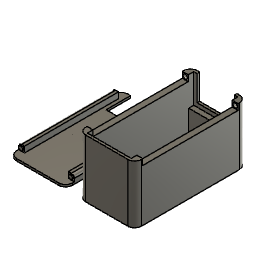
WirelessTouchLight v5 (Autodesk Fusion 360 design; units mm, degrees)
Autodesk Fusion 360 part; units mm, degrees
form "Form1" [no effect]
sketch "Bases" plane through (0, 0, 0) normal (0, 1, 0) x (1, 0, 0)
  line L0 (7.8348, -10.0405) -> (32.8348, -10.0405)
  line L1 (36.8348, -6.0405) -> (36.8348, 51.9595)
  line L2 (32.8348, 55.9595) -> (7.8348, 55.9595)
  line L3 (3.8348, 51.9595) -> (3.8348, -6.0405)
  arc A0 (7.8348, 55.9595) -> (3.8348, 51.9595) centre (7.8348, 51.9595) ccw
  arc A1 (36.8348, 51.9595) -> (32.8348, 55.9595) centre (32.8348, 51.9595) ccw
  arc A2 (32.8348, -10.0405) -> (36.8348, -6.0405) centre (32.8348, -6.0405) ccw
  arc A3 (3.8348, -6.0405) -> (7.8348, -10.0405) centre (7.8348, -6.0405) ccw
  arc A4 (3.8348, -6.0405) -> (7.8348, -10.0405) centre (7.8348, -6.0405) ccw
  arc A5 (32.8348, -10.0405) -> (36.8348, -6.0405) centre (32.8348, -6.0405) ccw
  line L4 (3.8348, 51.9595) -> (3.8348, -6.0405)
  line L5 (36.8348, -6.0405) -> (36.8348, 51.9595)
  line L6 (7.8348, -10.0405) -> (32.8348, -10.0405)
  arc A6 (7.8348, 55.9595) -> (3.8348, 51.9595) centre (7.8348, 51.9595) ccw
  line L7 (32.8348, 55.9595) -> (7.8348, 55.9595)
  arc A7 (36.8348, 51.9595) -> (32.8348, 55.9595) centre (32.8348, 51.9595) ccw
  line L8 (-37.5541, 52.4657) -> (-37.5541, -5.5343)
  arc A8 (-8.5541, -9.5343) -> (-4.5541, -5.5343) centre (-8.5541, -5.5343) ccw
  line L9 (-33.5541, -9.5343) -> (-8.5541, -9.5343)
  line L10 (-8.5541, 56.4657) -> (-33.5541, 56.4657)
  arc A9 (-33.5541, 56.4657) -> (-37.5541, 52.4657) centre (-33.5541, 52.4657) ccw
  arc A10 (-4.5541, 52.4657) -> (-8.5541, 56.4657) centre (-8.5541, 52.4657) ccw
  arc A11 (-37.5541, -5.5343) -> (-33.5541, -9.5343) centre (-33.5541, -5.5343) ccw
  line L11 (-4.5541, -5.5343) -> (-4.5541, 52.4657)
  line L12 (-37.5541, 51.2657) -> (-34.0541, 51.2657)
  line L13 (-34.0541, 51.2657) -> (-34.0541, -4.3343)
  line L14 (-34.0541, -4.3343) -> (-37.5541, -4.3343)
  line L15 (-37.5541, -4.3343) -> (-37.5541, 51.2657)
  line L16 (-4.5541, 51.2657) -> (-8.0541, 51.2657)
  line L17 (-8.0541, 51.2657) -> (-8.0541, -4.3343)
  line L18 (-8.0541, -4.3343) -> (-4.5541, -4.3343)
  line L19 (-4.5541, -4.3343) -> (-4.5541, 51.2657)
  dimension "d14" = 4
  dimension "d15" = 4
  dimension "d16" = 66
  dimension "d18" = 33
  dimension "d31" = 4
  dimension "d32" = 4
  dimension "d33" = 66
  dimension "d34" = 33
  dimension "d35" = 4
  dimension "d36" = 4
  dimension "d37" = 66
  dimension "d38" = 33
  dimension "d45" = 55.6
  dimension "d46" = 3.5
  dimension "d47" = 3.5
  constraint horizontal L0
  constraint vertical L1
  constraint horizontal L2
  constraint vertical L3
  constraint tangent L2 A0
  constraint tangent L3 A0
  constraint tangent L1 A1
  constraint tangent L2 A1
  constraint tangent L0 A2
  constraint tangent L1 A2
  constraint equal A1 A2
  constraint tangent L0 A3
  constraint tangent L3 A3
  constraint equal A1 A3
  constraint horizontal L6
  constraint vertical L5
  constraint horizontal L7
  constraint vertical L4
  constraint tangent A6 L7
  constraint tangent L4 A6
  constraint tangent L5 A7
  constraint tangent L7 A7
  constraint tangent A5 L6
  constraint tangent A5 L5
  constraint equal A5 A7
  constraint tangent A4 L6
  constraint tangent A4 L4
  constraint equal A4 A7
  constraint horizontal L9
  constraint vertical L11
  constraint horizontal L10
  constraint vertical L8
  constraint tangent L10 A9
  constraint tangent L8 A9
  constraint tangent A10 L11
  constraint tangent L10 A10
  constraint tangent A8 L9
  constraint tangent A8 L11
  constraint equal A8 A10
  constraint tangent L9 A11
  constraint tangent L8 A11
  constraint equal A10 A11
  constraint horizontal L12
  constraint vertical L13
  constraint horizontal L14
  constraint vertical L15
  constraint coincident L8 L12.start
  constraint midpoint L8 L15
  constraint horizontal L16
  constraint vertical L17
  constraint horizontal L18
  constraint vertical L19
  constraint collinear L12 L16
  constraint collinear L14 L18
  constraint collinear L11 L19
  measures "d14" radius of A0
  measures "d15" radius of A1
  measures "d16" distance of L0 L2
  measures "d18" distance of L1 L3
  measures "d31" radius of A6
  measures "d32" radius of A7
  measures "d33" distance of L6 L7
  measures "d34" distance of L4 L5
  measures "d35" radius of A9
  measures "d36" radius of A10
  measures "d37" distance of L9 L10
  measures "d38" distance of L8 L11
  measures "d45" distance of L12.end L13.end
  measures "d46" distance of L12.start L12.end
  measures "d47" distance of L16.start L16.end
extrude "WirelessTouchLight Box" add sketch "Bases" along normal blind 34.25 contours L0 L1 L2 L3 A0 A1 A2 A3 A4 A5 L4 L5 L6 A6 L7 A7 makes body 1
sketch "TopBox" plane through (0, 34.25, 0) normal (0, 1, 0) x (-1, 0, 0)
  arc A0 (-3.8348, 6.0405) -> (-7.8348, 10.0405) centre (-7.8348, 6.0405) ccw
  line L0 (-7.8348, 10.0405) -> (-32.8348, 10.0405)
  arc A1 (-32.8348, 10.0405) -> (-36.8348, 6.0405) centre (-32.8348, 6.0405) ccw
  line L1 (-36.8348, 6.0405) -> (-36.8348, -51.9595)
  arc A2 (-36.8348, -51.9595) -> (-32.8348, -55.9595) centre (-32.8348, -51.9595) ccw
  line L2 (-32.8348, -55.9595) -> (-7.8348, -55.9595)
  arc A3 (-7.8348, -55.9595) -> (-3.8348, -51.9595) centre (-7.8348, -51.9595) ccw
  line L3 (-3.8348, -51.9595) -> (-3.8348, 6.0405)
  line L4 (-7.3348, 8.5405) -> (-33.3348, 8.5405)
  line L5 (-33.3348, 8.5405) -> (-33.3348, -54.4595)
  line L6 (-33.3348, -54.4595) -> (-7.3348, -54.4595)
  line L7 (-7.3348, -54.4595) -> (-7.3348, 8.5405)
  line L8 (-3.8348, -51.1595) -> (-7.3348, -51.1595)
  line L9 (-7.3348, -51.1595) -> (-7.3348, 5.2405)
  line L10 (-7.3348, 5.2405) -> (-3.8348, 5.2405)
  line L11 (-3.8348, 5.2405) -> (-3.8348, -51.1595)
  line L12 (-33.3348, -51.1595) -> (-36.8348, -51.1595)
  line L13 (-36.8348, -51.1595) -> (-36.8348, 5.2405)
  line L14 (-36.8348, 5.2405) -> (-33.3348, 5.2405)
  line L15 (-33.3348, 5.2405) -> (-33.3348, -51.1595)
  dimension "d22" = 63
  dimension "d23" = 26
  dimension "d24" = 1.5
  dimension "d25" = 3.5
  dimension "d28" = 56.4
  constraint horizontal L4
  constraint vertical L5
  constraint horizontal L6
  constraint vertical L7
  constraint horizontal L8
  constraint vertical L9
  constraint horizontal L10
  constraint vertical L11
  constraint coincident L7 L9.end
  constraint coincident L3 L8.start
  constraint midpoint L3 L11
  constraint horizontal L12
  constraint vertical L13
  constraint horizontal L14
  constraint vertical L15
  constraint coincident L1 L13.end
  constraint coincident L5 L12.start
  constraint midpoint L1 L13
  constraint collinear L8 L12
  measures "d22" distance of L4.start L6.end
  measures "d23" distance of L4.start L4.end
  measures "d24" distance of L0 L4
  measures "d25" distance of L3 L7
  measures "d28" distance of L8.start L10.end
extrude "Extrude2" cut sketch "TopBox" against normal blind 33 contours L4 L5 L6 L7 L9 L15 bodies 1
extrude "Extrude3" cut sketch "TopBox" against normal blind 3.5 contours L3 L7 L8 L9 L10 L11 | L1 L5 L12 L13 L14 L15 bodies 1
extrude "Extrude4" add sketch "Bases" along normal blind 1.25 separate body contours L8 A8 L9 L10 A9 A10 A11 L11 L12 L13 L14 L16 L17 L18 | L8 L12 L13 L14 L15 | L11 L16 L17 L18 L19 makes body 2
extrude "Extrude5" add sketch "Bases" along normal blind 4.75 contours L8 L12 L13 L14 L15 | L11 L16 L17 L18 L19 bodies 2
fillet "Fillet1" radius 1.75 1 edges at (-4.5541, 4.75, -23.4657) on bodies 2
fillet "Fillet1" radius 1.75 1 edges at (-37.5541, 4.75, -23.4657) on bodies 2
sphere "SpherePrimitive10" cut diameter 2.5 placed x (1, 0, 0) y (0, 1, 0) z (0, 0, 1) at (35.0848, 32.5, -51.1595) bodies 1
pattern_linear "R-Pattern1" count 2 spacing 56.4 along (0, 0, 1) count 2 spacing 29.5 along (-1, 0, 0) of "SpherePrimitive10"
sphere "SpherePrimitive9" add diameter 2.5 placed x (-1, 0, 0) y (0, 1, 0) z (0, 0, -1) at (-6.3041, 3, -51.2657) bodies 2
pattern_linear "R-Pattern2" count 2 spacing 55.6 along (0, 0, 1) count 2 spacing 29.5 along (-1, 0, 0) of "SpherePrimitive9"
sketch "CutSpheres" plane through (0, 1.25, 0) normal (0, 1, 0) x (-1, 0, 0)
  line L0 (8.0541, -51.2657) -> (4.5541, -51.2657)
  line L1 (4.5541, -51.2657) -> (4.5541, -52.4657)
  arc A0 (4.5541, -52.4657) -> (8.5541, -56.4657) centre (8.5541, -52.4657) ccw
  line L2 (8.5541, -56.4657) -> (33.5541, -56.4657)
  arc A1 (33.5541, -56.4657) -> (37.5541, -52.4657) centre (33.5541, -52.4657) ccw
  line L3 (37.5541, -52.4657) -> (37.5541, -51.2657)
  line L4 (37.5541, -51.2657) -> (34.0541, -51.2657)
  line L5 (34.0541, -51.2657) -> (34.0541, 4.3343)
  line L6 (34.0541, 4.3343) -> (37.5541, 4.3343)
  line L7 (37.5541, 4.3343) -> (37.5541, 5.5343)
  arc A2 (37.5541, 5.5343) -> (33.5541, 9.5343) centre (33.5541, 5.5343) ccw
  line L8 (33.5541, 9.5343) -> (8.5541, 9.5343)
  arc A3 (8.5541, 9.5343) -> (4.5541, 5.5343) centre (8.5541, 5.5343) ccw
  line L9 (4.5541, 5.5343) -> (4.5541, 4.3343)
  line L10 (4.5541, 4.3343) -> (8.0541, 4.3343)
  line L11 (8.0541, 4.3343) -> (8.0541, -51.2657)
  line L12 (7.5541, -52.5157) -> (5.0541, -52.5157)
  line L13 (5.0541, -52.5157) -> (5.0541, -51.8157)
  line L14 (5.0541, -51.8157) -> (7.5541, -51.8157)
  line L15 (7.5541, -51.8157) -> (7.5541, -52.5157)
  line L16 (4.5541, 5.5343) -> (4.5541, -52.4657)
  line L17 (4.5541, -51.2657) -> (8.0541, -51.2657)
  line L18 (7.5541, 4.8843) -> (5.0541, 4.8843)
  line L19 (5.0541, 4.8843) -> (5.0541, 5.5843)
  line L20 (5.0541, 5.5843) -> (7.5541, 5.5843)
  line L21 (7.5541, 5.5843) -> (7.5541, 4.8843)
  line L22 (37.0541, 4.8843) -> (34.5541, 4.8843)
  line L23 (34.5541, 4.8843) -> (34.5541, 5.5843)
  line L24 (34.5541, 5.5843) -> (37.0541, 5.5843)
  line L25 (37.0541, 5.5843) -> (37.0541, 4.8843)
  line L26 (37.0541, -52.5157) -> (34.5541, -52.5157)
  line L27 (34.5541, -52.5157) -> (34.5541, -51.8157)
  line L28 (34.5541, -51.8157) -> (37.0541, -51.8157)
  line L29 (37.0541, -51.8157) -> (37.0541, -52.5157)
  line L30 (8.0541, 4.3343) -> (4.5541, 4.3343)
  line L31 (34.0541, 4.3343) -> (37.5541, 4.3343)
  line L32 (37.5541, -51.2657) -> (34.0541, -51.2657)
  line L33 (37.5541, -52.4657) -> (37.5541, 5.5343)
  dimension "d71" = 0.5
  dimension "d72" = 2.5
  dimension "d73" = 0.55
  dimension "d74" = 0.7
  dimension "d77" = 0.55
  dimension "d78" = 0.55
  dimension "d79" = 0.55
  dimension "d80" = 0.7
  dimension "d81" = 0.7
  dimension "d82" = 0.7
  dimension "d83" = 0.5
  dimension "d84" = 0.5
  dimension "d85" = 0.5
  dimension "d86" = 2.5
  dimension "d87" = 2.5
  dimension "d88" = 2.5
  constraint horizontal L12
  constraint vertical L13
  constraint horizontal L14
  constraint vertical L15
  constraint horizontal L18
  constraint vertical L19
  constraint horizontal L20
  constraint vertical L21
  constraint horizontal L22
  constraint vertical L23
  constraint horizontal L24
  constraint vertical L25
  constraint horizontal L26
  constraint vertical L27
  constraint horizontal L28
  constraint vertical L29
  measures "d71" distance of L13 L16
  measures "d72" distance of L12.start L12.end
  measures "d73" distance of L14 L17
  measures "d74" distance of L12.end L13.end
  measures "d77" distance of L18 L30
  measures "d78" distance of L22 L31
  measures "d79" distance of L28 L32
  measures "d80" distance of L18.end L19.end
  measures "d81" distance of L22.start L24.end
  measures "d82" distance of L26.start L28.end
  measures "d83" distance of L16 L19
  measures "d84" distance of L25 L33
  measures "d85" distance of L29 L33
  measures "d86" distance of L26.start L26.end
  measures "d87" distance of L23.end L24.end
  measures "d88" distance of L19.end L20.end
extrude "Extrude6" cut sketch "CutSpheres" along normal blind 3 contours L12 L13 L14 L15 | L18 L19 L20 L21 | L22 L23 L24 L25 | L26 L27 L28 L29 bodies 2
sketch "Supports" plane through (0, 1.25, 0) normal (0, 1, 0) x (-1, 0, 0)
  line L0 (-7.3348, -54.4595) -> (-7.3348, 8.5405)
  line L1 (-7.3348, 8.5405) -> (-33.3348, 8.5405)
  line L2 (-33.3348, 8.5405) -> (-33.3348, -54.4595)
  line L3 (-33.3348, -54.4595) -> (-7.3348, -54.4595)
  line L4 (-11.3348, -20.0595) -> (-33.3348, -20.0595)
  line L5 (-33.3348, -20.0595) -> (-33.3348, -26.0595)
  line L6 (-33.3348, -26.0595) -> (-11.3348, -26.0595)
  line L7 (-11.3348, -26.0595) -> (-11.3348, -20.0595)
  line L8 (-7.3348, 2.5405) -> (-10.3348, 2.5405)
  line L9 (-10.3348, 2.5405) -> (-10.3348, 8.5405)
  line L10 (-10.3348, 8.5405) -> (-7.3348, 8.5405)
  line L11 (-7.3348, 8.5405) -> (-7.3348, 2.5405)
  line L12 (-33.3348, 2.5405) -> (-30.3348, 2.5405)
  line L13 (-30.3348, 2.5405) -> (-30.3348, 8.5405)
  line L14 (-30.3348, 8.5405) -> (-33.3348, 8.5405)
  line L15 (-33.3348, 8.5405) -> (-33.3348, 2.5405)
  line L16 (-7.3348, -54.4595) -> (-33.3348, -54.4595)
  line L17 (-33.3348, -54.4595) -> (-33.3348, -51.4595)
  line L18 (-33.3348, -51.4595) -> (-7.3348, -51.4595)
  line L19 (-7.3348, -51.4595) -> (-7.3348, -54.4595)
  dimension "d93" = 6
  dimension "d94" = 22
  dimension "d95" = 6
  dimension "d96" = 6
  dimension "d97" = 3
  dimension "d98" = 3
  dimension "d141" = 3
  dimension "d146" = 28.6
  constraint horizontal L4
  constraint vertical L5
  constraint horizontal L6
  constraint vertical L7
  constraint horizontal L8
  constraint vertical L9
  constraint horizontal L10
  constraint vertical L11
  constraint horizontal L12
  constraint vertical L13
  constraint horizontal L14
  constraint vertical L15
  constraint coincident L0 L8.start
  constraint coincident L2 L12.start
  constraint horizontal L16
  constraint vertical L17
  constraint horizontal L18
  constraint vertical L19
  constraint coincident L2 L17.end
  constraint coincident L0.start L16
  constraint coincident L0.end L10
  constraint coincident L1.end L14
  constraint coincident L2 L4.end
  measures "d93" distance of L4.end L5.end
  measures "d94" distance of L5.end L6.end
  measures "d95" distance of L8.end L9.end
  measures "d96" distance of L12.end L13.end
  measures "d97" distance of L8.start L8.end
  measures "d98" distance of L12.start L12.end
  measures "d141" distance of L16 L18
  measures "d146" distance of L4 L10
extrude "Extrude7" add sketch "Supports" along normal blind 3 contours L0 L1 L8 L9 L10 L11 | L2 L4 L5 L6 L7 | L1 L2 L12 L13 L14 L15 bodies 1
extrude "Extrude14" add sketch "Supports" along normal blind 15.75 contours L0 L2 L3 L16 L17 L18 L19 bodies 1
sketch "BornierHole" plane through (0, 0, -55.9595) normal (0, 0, -1) x (-1, 0, 0)
  line L0 (-32.8348, 0) -> (-7.8348, 0)
  line L1 (-7.8348, 0) -> (-7.8348, 34.25)
  line L2 (-7.8348, 34.25) -> (-32.8348, 34.25)
  line L3 (-32.8348, 34.25) -> (-32.8348, 0)
  line L4 (-31.3348, 34.25) -> (-9.3348, 34.25)
  line L5 (-9.3348, 34.25) -> (-9.3348, 19.25)
  line L6 (-9.3348, 19.25) -> (-31.3348, 19.25)
  line L7 (-31.3348, 19.25) -> (-31.3348, 34.25)
  dimension "d116" = 22
  dimension "d144" = 15
  constraint horizontal L4
  constraint vertical L5
  constraint horizontal L6
  constraint vertical L7
  constraint coincident L2 L4.start
  constraint midpoint L2 L4
  measures "d116" distance of L4.start L4.end
  measures "d144" distance of L4 L6
extrude "Extrude10" cut sketch "BornierHole" against normal blind 1.5 contours L2 L4 L5 L6 L7 bodies 1
sketch "BordnierHoleAndMaintainLeg" plane through (0, 1.25, 0) normal (0, 1, 0) x (-1, 0, 0)
  line L0 (8.0541, -51.2657) -> (4.5541, -51.2657)
  line L1 (4.5541, -51.2657) -> (4.5541, -52.4657)
  arc A0 (4.5541, -52.4657) -> (8.5541, -56.4657) centre (8.5541, -52.4657) ccw
  line L2 (8.5541, -56.4657) -> (33.5541, -56.4657)
  arc A1 (33.5541, -56.4657) -> (37.5541, -52.4657) centre (33.5541, -52.4657) ccw
  line L3 (37.5541, -52.4657) -> (37.5541, -51.2657)
  line L4 (37.5541, -51.2657) -> (34.0541, -51.2657)
  line L5 (34.0541, -51.2657) -> (34.0541, 4.3343)
  line L6 (34.0541, 4.3343) -> (37.5541, 4.3343)
  line L7 (37.5541, 4.3343) -> (37.5541, 5.5343)
  arc A2 (37.5541, 5.5343) -> (33.5541, 9.5343) centre (33.5541, 5.5343) ccw
  line L8 (33.5541, 9.5343) -> (8.5541, 9.5343)
  arc A3 (8.5541, 9.5343) -> (4.5541, 5.5343) centre (8.5541, 5.5343) ccw
  line L9 (4.5541, 5.5343) -> (4.5541, 4.3343)
  line L10 (4.5541, 4.3343) -> (8.0541, 4.3343)
  line L11 (8.0541, 4.3343) -> (8.0541, -51.2657)
  line L12 (32.0541, -56.4657) -> (10.0541, -56.4657)
  line L13 (10.0541, -56.4657) -> (10.0541, -41.9657)
  line L14 (10.0541, -41.9657) -> (32.0541, -41.9657)
  line L15 (32.0541, -41.9657) -> (32.0541, -56.4657)
  dimension "d120" = 22
  dimension "d121" = 14.5
  constraint horizontal L12
  constraint vertical L13
  constraint horizontal L14
  constraint vertical L15
  constraint coincident L2 L12.start
  constraint midpoint L2 L12
  measures "d120" distance of L12.start L12.end
  measures "d121" distance of L12.start L14.end
extrude "Extrude11" cut sketch "BordnierHoleAndMaintainLeg" against normal blind 1.25 contours L2 L12 L13 L14 L15 bodies 2
sketch "ModuleName" plane through (0, 0, 0) normal (0, -1, 0) x (1, 0, 0)
  line L0 (-32.0541, -56.4657) -> (-32.0541, -41.9657)
  line L1 (-32.0541, -41.9657) -> (-10.0541, -41.9657)
  line L2 (-10.0541, -41.9657) -> (-10.0541, -56.4657)
  line L3 (-10.0541, -56.4657) -> (-8.5541, -56.4657)
  arc A0 (-8.5541, -56.4657) -> (-4.5541, -52.4657) centre (-8.5541, -52.4657) ccw
  line L4 (-4.5541, -52.4657) -> (-4.5541, 5.5343)
  arc A1 (-4.5541, 5.5343) -> (-8.5541, 9.5343) centre (-8.5541, 5.5343) ccw
  line L5 (-8.5541, 9.5343) -> (-33.5541, 9.5343)
  arc A2 (-33.5541, 9.5343) -> (-37.5541, 5.5343) centre (-33.5541, 5.5343) ccw
  line L6 (-37.5541, 5.5343) -> (-37.5541, -52.4657)
  arc A3 (-37.5541, -52.4657) -> (-33.5541, -56.4657) centre (-33.5541, -52.4657) ccw
  line L7 (-33.5541, -56.4657) -> (-32.0541, -56.4657)
  line L8 (-8.3337, -24.7187) -> (-33.0602, -24.7187) construction
  line L9 (-33.0602, -24.7187) -> (-33.0602, -29.7187) construction
  line L10 (-33.0602, -29.7187) -> (-8.3337, -29.7187) construction
  line L11 (-8.3337, -29.7187) -> (-8.3337, -24.7187) construction
  line L12 (-10.3438, -18.9177) -> (-30.6074, -18.9177) construction
  line L13 (-30.6074, -18.9177) -> (-30.6074, -23.9177) construction
  line L14 (-30.6074, -23.9177) -> (-10.3438, -23.9177) construction
  line L15 (-10.3438, -23.9177) -> (-10.3438, -18.9177) construction
  line L16 (-15.3778, -7.1463) -> (-25.4193, -7.1463) construction
  line L17 (-25.4193, -7.1463) -> (-25.4193, -12.1463) construction
  line L18 (-25.4193, -12.1463) -> (-15.3778, -12.1463) construction
  line L19 (-15.3778, -12.1463) -> (-15.3778, -7.1463) construction
  line L20 (-7.7862, -12.9218) -> (-34.461, -12.9218) construction
  line L21 (-34.461, -12.9218) -> (-34.461, -17.9218) construction
  line L22 (-34.461, -17.9218) -> (-7.7862, -17.9218) construction
  line L23 (-7.7862, -17.9218) -> (-7.7862, -12.9218) construction
  line L24 (-10.1628, -34.4794) -> (-14.237, -34.4794) construction
  line L25 (-14.237, -34.4794) -> (-14.237, -41.4794) construction
  line L26 (-14.237, -41.4794) -> (-10.1628, -41.4794) construction
  line L27 (-10.1628, -41.4794) -> (-10.1628, -34.4794) construction
  line L28 (-28.4269, -34.6057) -> (-31.9542, -34.6057) construction
  line L29 (-31.9542, -34.6057) -> (-31.9542, -41.6057) construction
  line L30 (-31.9542, -41.6057) -> (-28.4269, -41.6057) construction
  line L31 (-28.4269, -41.6057) -> (-28.4269, -34.6057) construction
  line L32 (-22.5488, -34.6057) -> (-28.6395, -34.6057) construction
  line L33 (-28.6395, -34.6057) -> (-28.6395, -41.6057) construction
  line L34 (-28.6395, -41.6057) -> (-22.5488, -41.6057) construction
  line L35 (-22.5488, -41.6057) -> (-22.5488, -34.6057) construction
  line L36 (-15.9454, -34.4754) -> (-20.8057, -34.4754) construction
  line L37 (-20.8057, -34.4754) -> (-20.8057, -41.4754) construction
  line L38 (-20.8057, -41.4754) -> (-15.9454, -41.4754) construction
  line L39 (-15.9454, -41.4754) -> (-15.9454, -34.4754) construction
  text T0 "DomoChip" font "Arial" height 5 bold align ink ink in box 0 x 0 at (-8.3337, -24.7187) x (-1, 0) y (0, -1) spacing 1 kerned height is em
  text T1 "Wireless" font "Arial" height 5 bold align ink ink in box 0 x 0 at (-10.3438, -18.9177) x (-1, 0) y (0, -1) spacing 1 kerned height is em
  text T2 "TouchLight" font "Arial" height 5 bold align ink ink in box 0 x 0 at (-7.7862, -12.9218) x (-1, 0) y (0, -1) spacing 1 kerned height is em
  text T3 "V1.0" font "Arial" height 5 bold align ink ink in box 0 x 0 at (-15.3778, -7.1463) x (-1, 0) y (0, -1) spacing 1 kerned height is em
  text T4 "L" font "Arial" height 7 bold align ink ink in box 0 x 0 at (-28.4269, -34.6057) x (-1, 0) y (0, -1) spacing 1 kerned height is em
  text T5 "S" font "Arial" height 7 bold align ink ink in box 0 x 0 at (-10.1628, -34.4794) x (-1, 0) y (0, -1) spacing 1 kerned height is em
  text T6 "N" font "Arial" height 7 bold align ink ink in box 0 x 0 at (-22.5488, -34.6057) x (-1, 0) y (0, -1) spacing 1 kerned height is em
  text T7 "O" font "Arial" height 7 bold align ink ink in box 0 x 0 at (-15.9454, -34.4754) x (-1, 0) y (0, -1) spacing 1 kerned height is em
  constraint perpendicular L8 L9
  constraint parallel L8 L10
  constraint parallel L9 L11
  constraint perpendicular L12 L13
  constraint parallel L12 L14
  constraint parallel L13 L15
  constraint perpendicular L16 L17
  constraint parallel L16 L18
  constraint parallel L17 L19
  constraint perpendicular L20 L21
  constraint parallel L20 L22
  constraint parallel L21 L23
  constraint perpendicular L24 L25
  constraint parallel L24 L26
  constraint parallel L25 L27
  constraint perpendicular L28 L29
  constraint parallel L28 L30
  constraint parallel L29 L31
  constraint perpendicular L32 L33
  constraint parallel L32 L34
  constraint parallel L33 L35
  constraint perpendicular L36 L37
  constraint parallel L36 L38
  constraint parallel L37 L39
extrude "Extrude13" cut sketch "ModuleName" against normal blind 0.5 text T0 T1 T2 T3 T5 T4 T7 T6 bodies 2
equation "_width = 63 mm" comment "width of the box (affects the length of the hinges)"
equation "_length = 26 mm" comment "length of the box"
equation "_height = 33 mm" comment "height of the box"
equation "_rounding = 4 mm" comment "rounding radius of the corners of the box"
equation "_minimumWallThickness = 0.5 mm" comment "thickness of the walls around the magnets"
equation "_sidewallThickness = 1.5 mm" comment "thickness of the side walls without the hinge"
equation "_horizontalThickness = 1.25 mm" comment "thickness of the bottom of the box or the top of the lid"
equation "_magnetDiameter = 2.5 mm" comment "diameter of magnets in the hinge"
equation "_magnetHeight = 1 mm" comment "height magnets in the hinge"
equation "_hingeGap = 0.4 mm" comment "gap bewteen the lid and box parts"
equation "_hingeOverlap = 0.15 mm" comment "Size of lid's spheres that go into box holes"
equation "d14 = _rounding"
equation "d15 = _rounding"
equation "d16 = _width + 2 * _sidewallThickness"
equation "d18 = _length + 4 * _minimumWallThickness + 2 * _magnetDiameter"
equation "d20 = _height + _horizontalThickness"
equation "d22 = _width"
equation "d23 = _length"
equation "d24 = _sidewallThickness"
equation "d25 = 2 * _minimumWallThickness + _magnetDiameter"
equation "d26 = -_height"
equation "d28 = _width + 2 * _sidewallThickness - 2 * _rounding - 2 * _magnetHeight + _hingeGap"
equation "d29 = -_magnetDiameter - 2 * _minimumWallThickness"
equation "d31 = _rounding"
equation "d32 = _rounding"
equation "d33 = _width + 2 * _sidewallThickness"
equation "d34 = _length + 4 * _minimumWallThickness + 2 * _magnetDiameter"
equation "d35 = _rounding"
equation "d36 = _rounding"
equation "d37 = _width + 2 * _sidewallThickness"
equation "d38 = _length + 4 * _minimumWallThickness + 2 * _magnetDiameter"
equation "d43 = _horizontalThickness"
equation "d45 = _width + 2 * _sidewallThickness - 2 * _rounding - 2 * _magnetHeight - _hingeGap"
equation "d46 = _magnetDiameter + 2 * _minimumWallThickness"
equation "d47 = _magnetDiameter + 2 * _minimumWallThickness"
equation "d48 = _horizontalThickness + _magnetDiameter + 2 * _minimumWallThickness"
equation "d50 = ( _magnetDiameter + 2 * _minimumWallThickness ) / 2"
equation "d51 = ( _magnetDiameter + 2 * _minimumWallThickness ) / 2"
equation "d59 = _width + 2 * _sidewallThickness - 2 * _rounding - 2 * _magnetHeight + _hingeGap"
equation "d60 = -_length - _magnetDiameter - 2 * _minimumWallThickness"
equation "d64 = _width + 2 * _sidewallThickness - 2 * _rounding - 2 * _magnetHeight - _hingeGap"
equation "d65 = -_length - _magnetDiameter - 2 * _minimumWallThickness"
equation "d71 = _minimumWallThickness"
equation "d72 = _magnetDiameter"
equation "d73 = _hingeGap + _hingeOverlap"
equation "d74 = _magnetDiameter / 2 - _hingeGap - _hingeOverlap"
equation "d75 = _minimumWallThickness + _magnetDiameter"
equation "d77 = _hingeGap + _hingeOverlap"
equation "d78 = _hingeGap + _hingeOverlap"
equation "d79 = _hingeGap + _hingeOverlap"
equation "d80 = _magnetDiameter / 2 - _hingeGap - _hingeOverlap"
equation "d81 = _magnetDiameter / 2 - _hingeGap - _hingeOverlap"
equation "d82 = _magnetDiameter / 2 - _hingeGap - _hingeOverlap"
equation "d83 = _minimumWallThickness"
equation "d84 = _minimumWallThickness"
equation "d85 = _minimumWallThickness"
equation "d86 = _magnetDiameter"
equation "d87 = _magnetDiameter"
equation "d88 = _magnetDiameter"
equation "d118 = -_sidewallThickness"
equation "d121 = 13 mm + _sidewallThickness"
equation "d127 = -_horizontalThickness"
equation "d137 = _magnetDiameter"
equation "d145 = _magnetDiameter"
named bodies: "WirelessTouchLight Box", "WirelessTouchLight Lid"
